Autodesk Inventor part; units mm, degrees
(part 4 of 4)
  line L2671 (9.6574, 16.9003) -> (9.6038, 16.7112)
  line L2672 (9.6038, 16.7112) -> (9.5545, 16.5545)
  line L2673 (9.5545, 16.5545) -> (9.5433, 16.503)
  line L2674 (9.5433, 16.503) -> (9.5383, 16.4584)
  line L2675 (9.5383, 16.4584) -> (9.5392, 16.4209)
  line L2676 (9.5392, 16.4209) -> (9.5457, 16.3908)
  line L2677 (9.5457, 16.3908) -> (9.5575, 16.3682)
  line L2678 (9.5575, 16.3682) -> (9.5743, 16.3534)
  line L2679 (9.5743, 16.3534) -> (9.6034, 16.3364)
  line L2680 (9.6034, 16.3364) -> (9.9014, 16.1575)
  line L2681 (9.9014, 16.1575) -> (10.196, 15.9733)
  line L2682 (10.196, 15.9733) -> (10.2244, 15.9551)
  line L2683 (10.2244, 15.9551) -> (10.2452, 15.9468)
  line L2684 (10.2452, 15.9468) -> (10.2706, 15.9466)
  line L2685 (10.2706, 15.9466) -> (10.3004, 15.9544)
  line L2686 (10.3004, 15.9544) -> (10.3342, 15.9707)
  line L2687 (10.3342, 15.9707) -> (10.3717, 15.9954)
  line L2688 (10.3717, 15.9954) -> (10.4125, 16.0287)
  line L2689 (10.4125, 16.0287) -> (10.5298, 16.1438)
  line L2690 (10.5298, 16.1438) -> (10.6739, 16.2774)
  line L2691 (10.6739, 16.2774) -> (10.8486, 16.4262)
  line L2692 (10.8486, 16.4262) -> (11.0549, 16.5875)
  line L2693 (11.0549, 16.5875) -> (11.2943, 16.7591)
  line L2694 (11.2943, 16.7591) -> (11.4265, 16.8478)
  line L2695 (11.4265, 16.8478) -> (11.5685, 16.9387)
  line L2696 (11.5685, 16.9387) -> (11.7175, 17.0299)
  line L2697 (11.7175, 17.0299) -> (11.8785, 17.1238)
  line L2698 (11.8785, 17.1238) -> (12.0338, 17.2101)
  arc A76 (12.6491, 16.763) -> (12.0338, 17.2101) centre (0, 0) ccw
  line L2699 (12.6491, 16.763) -> (12.615, 16.5887)
  line L2700 (12.615, 16.5887) -> (12.5755, 16.4066)
  line L2701 (12.5755, 16.4066) -> (12.5348, 16.2367)
  line L2702 (12.5348, 16.2367) -> (12.4922, 16.0735)
  line L2703 (12.4922, 16.0735) -> (12.4487, 15.9204)
  line L2704 (12.4487, 15.9204) -> (12.3595, 15.6397)
  line L2705 (12.3595, 15.6397) -> (12.2698, 15.3936)
  line L2706 (12.2698, 15.3936) -> (12.1823, 15.1815)
  line L2707 (12.1823, 15.1815) -> (12.0998, 15.0031)
  line L2708 (12.0998, 15.0031) -> (12.0266, 14.856)
  line L2709 (12.0266, 14.856) -> (12.0075, 14.8069)
  line L2710 (12.0075, 14.8069) -> (11.9956, 14.7636)
  line L2711 (11.9956, 14.7636) -> (11.9906, 14.7264)
  line L2712 (11.9906, 14.7264) -> (11.9923, 14.6957)
  line L2713 (11.9923, 14.6957) -> (12.0004, 14.6716)
  line L2714 (12.0004, 14.6716) -> (12.0147, 14.6544)
  line L2715 (12.0147, 14.6544) -> (12.0408, 14.633)
  line L2716 (12.0408, 14.633) -> (12.307, 14.4097)
  line L2717 (12.307, 14.4097) -> (12.5693, 14.1816)
  line L2718 (12.5693, 14.1816) -> (12.5944, 14.1592)
  line L2719 (12.5944, 14.1592) -> (12.6137, 14.1478)
  line L2720 (12.6137, 14.1478) -> (12.6388, 14.1436)
  line L2721 (12.6388, 14.1436) -> (12.6694, 14.1467)
  line L2722 (12.6694, 14.1467) -> (12.7053, 14.1574)
  line L2723 (12.7053, 14.1574) -> (12.7462, 14.1759)
  line L2724 (12.7462, 14.1759) -> (12.7918, 14.2025)
  line L2725 (12.7918, 14.2025) -> (12.9256, 14.2978)
  line L2726 (12.9256, 14.2978) -> (13.0888, 14.4072)
  line L2727 (13.0888, 14.4072) -> (13.2846, 14.5269)
  line L2728 (13.2846, 14.5269) -> (13.5137, 14.6539)
  line L2729 (13.5137, 14.6539) -> (13.777, 14.786)
  line L2730 (13.777, 14.786) -> (13.9214, 14.8528)
  line L2731 (13.9214, 14.8528) -> (14.0759, 14.9205)
  line L2732 (14.0759, 14.9205) -> (14.2373, 14.9872)
  line L2733 (14.2373, 14.9872) -> (14.411, 15.0547)
  line L2734 (14.411, 15.0547) -> (14.5779, 15.1157)
  arc A77 (15.1157, 14.5779) -> (14.5779, 15.1157) centre (0, 0) ccw
  line L2735 (15.1157, 14.5779) -> (15.0547, 14.411)
  line L2736 (15.0547, 14.411) -> (14.9872, 14.2373)
  line L2737 (14.9872, 14.2373) -> (14.9205, 14.0759)
  line L2738 (14.9205, 14.0759) -> (14.8529, 13.9214)
  line L2739 (14.8529, 13.9214) -> (14.786, 13.777)
  line L2740 (14.786, 13.777) -> (14.654, 13.5137)
  line L2741 (14.654, 13.5137) -> (14.5269, 13.2846)
  line L2742 (14.5269, 13.2846) -> (14.4072, 13.0888)
  line L2743 (14.4072, 13.0888) -> (14.2978, 12.9256)
  line L2744 (14.2978, 12.9256) -> (14.2025, 12.7918)
  line L2745 (14.2025, 12.7918) -> (14.1759, 12.7462)
  line L2746 (14.1759, 12.7462) -> (14.1574, 12.7053)
  line L2747 (14.1574, 12.7053) -> (14.1467, 12.6694)
  line L2748 (14.1467, 12.6694) -> (14.1436, 12.6387)
  line L2749 (14.1436, 12.6387) -> (14.1478, 12.6137)
  line L2750 (14.1478, 12.6137) -> (14.1592, 12.5944)
  line L2751 (14.1592, 12.5944) -> (14.1816, 12.5693)
  line L2752 (14.1816, 12.5693) -> (14.4097, 12.307)
  line L2753 (14.4097, 12.307) -> (14.633, 12.0408)
  line L2754 (14.633, 12.0408) -> (14.6544, 12.0147)
  line L2755 (14.6544, 12.0147) -> (14.6716, 12.0004)
  line L2756 (14.6716, 12.0004) -> (14.6957, 11.9923)
  line L2757 (14.6957, 11.9923) -> (14.7265, 11.9906)
  line L2758 (14.7265, 11.9906) -> (14.7636, 11.9956)
  line L2759 (14.7636, 11.9956) -> (14.8069, 12.0075)
  line L2760 (14.8069, 12.0075) -> (14.856, 12.0266)
  line L2761 (14.856, 12.0266) -> (15.0031, 12.0998)
  line L2762 (15.0031, 12.0998) -> (15.1815, 12.1823)
  line L2763 (15.1815, 12.1823) -> (15.3936, 12.2698)
  line L2764 (15.3936, 12.2698) -> (15.6397, 12.3595)
  line L2765 (15.6397, 12.3595) -> (15.9204, 12.4487)
  line L2766 (15.9204, 12.4487) -> (16.0735, 12.4922)
  line L2767 (16.0735, 12.4922) -> (16.2367, 12.5348)
  line L2768 (16.2367, 12.5348) -> (16.4066, 12.5755)
  line L2769 (16.4066, 12.5755) -> (16.5887, 12.615)
  line L2770 (16.5887, 12.615) -> (16.7631, 12.6491)
  arc A78 (17.2101, 12.0338) -> (16.7631, 12.6491) centre (0, 0) ccw
  line L2771 (17.2101, 12.0338) -> (17.1238, 11.8785)
  line L2772 (17.1238, 11.8785) -> (17.0299, 11.7175)
  line L2773 (17.0299, 11.7175) -> (16.9387, 11.5685)
  line L2774 (16.9387, 11.5685) -> (16.8478, 11.4265)
  line L2775 (16.8478, 11.4265) -> (16.7591, 11.2943)
  line L2776 (16.7591, 11.2943) -> (16.5875, 11.0549)
  line L2777 (16.5875, 11.0549) -> (16.4262, 10.8486)
  line L2778 (16.4262, 10.8486) -> (16.2774, 10.6739)
  line L2779 (16.2774, 10.6739) -> (16.1438, 10.5298)
  line L2780 (16.1438, 10.5298) -> (16.0287, 10.4125)
  line L2781 (16.0287, 10.4125) -> (15.9954, 10.3717)
  line L2782 (15.9954, 10.3717) -> (15.9707, 10.3342)
  line L2783 (15.9707, 10.3342) -> (15.9544, 10.3004)
  line L2784 (15.9544, 10.3004) -> (15.9466, 10.2706)
  line L2785 (15.9466, 10.2706) -> (15.9468, 10.2452)
  line L2786 (15.9468, 10.2452) -> (15.9551, 10.2244)
  line L2787 (15.9551, 10.2244) -> (15.9733, 10.196)
  line L2788 (15.9733, 10.196) -> (16.1575, 9.9013)
  line L2789 (16.1575, 9.9013) -> (16.3364, 9.6034)
  line L2790 (16.3364, 9.6034) -> (16.3535, 9.5743)
  line L2791 (16.3535, 9.5743) -> (16.3682, 9.5575)
  line L2792 (16.3682, 9.5575) -> (16.3908, 9.5457)
  line L2793 (16.3908, 9.5457) -> (16.4209, 9.5392)
  line L2794 (16.4209, 9.5392) -> (16.4584, 9.5383)
  line L2795 (16.4584, 9.5383) -> (16.503, 9.5433)
  line L2796 (16.503, 9.5433) -> (16.5545, 9.5545)
  line L2797 (16.5545, 9.5545) -> (16.7112, 9.6038)
  line L2798 (16.7112, 9.6038) -> (16.9003, 9.6574)
  line L2799 (16.9003, 9.6574) -> (17.1235, 9.7107)
  line L2800 (17.1235, 9.7107) -> (17.3806, 9.7608)
  line L2801 (17.3806, 9.7608) -> (17.6718, 9.805)
  line L2802 (17.6718, 9.805) -> (17.8299, 9.8239)
  line L2803 (17.8299, 9.8239) -> (17.9976, 9.8405)
  line L2804 (17.9976, 9.8405) -> (18.1718, 9.8541)
  line L2805 (18.1718, 9.8541) -> (18.3579, 9.8646)
  line L2806 (18.3579, 9.8646) -> (18.5354, 9.8711)
  arc A79 (18.8807, 9.1934) -> (18.5354, 9.8711) centre (0, 0) ccw
  line L2807 (18.8807, 9.1934) -> (18.7712, 9.0535)
  line L2808 (18.7712, 9.0535) -> (18.6532, 8.9092)
  line L2809 (18.6532, 8.9092) -> (18.5399, 8.7763)
  line L2810 (18.5399, 8.7763) -> (18.4279, 8.6503)
  line L2811 (18.4279, 8.6503) -> (18.3196, 8.5336)
  line L2812 (18.3196, 8.5336) -> (18.1127, 8.3239)
  line L2813 (18.1127, 8.3239) -> (17.9211, 8.1454)
  line L2814 (17.9211, 8.1454) -> (17.7468, 7.9961)
  line L2815 (17.7468, 7.9961) -> (17.5923, 7.8747)
  line L2816 (17.5923, 7.8747) -> (17.4603, 7.7769)
  line L2817 (17.4603, 7.7769) -> (17.4209, 7.7418)
  line L2818 (17.4209, 7.7418) -> (17.3907, 7.7086)
  line L2819 (17.3907, 7.7086) -> (17.3694, 7.6778)
  line L2820 (17.3694, 7.6778) -> (17.3569, 7.6496)
  line L2821 (17.3569, 7.6496) -> (17.3532, 7.6244)
  line L2822 (17.3532, 7.6244) -> (17.3581, 7.6026)
  line L2823 (17.3581, 7.6026) -> (17.3717, 7.5717)
  line L2824 (17.3717, 7.5717) -> (17.5075, 7.2518)
  line L2825 (17.5075, 7.2518) -> (17.6376, 6.9296)
  line L2826 (17.6376, 6.9296) -> (17.6499, 6.8982)
  line L2827 (17.6499, 6.8982) -> (17.6618, 6.8793)
  line L2828 (17.6618, 6.8793) -> (17.6823, 6.8641)
  line L2829 (17.6823, 6.8641) -> (17.711, 6.853)
  line L2830 (17.711, 6.853) -> (17.7479, 6.8462)
  line L2831 (17.7479, 6.8462) -> (17.7927, 6.8442)
  line L2832 (17.7927, 6.8442) -> (17.8454, 6.8472)
  line L2833 (17.8454, 6.8472) -> (18.0079, 6.8714)
  line L2834 (18.0079, 6.8714) -> (18.203, 6.8947)
  line L2835 (18.203, 6.8947) -> (18.4318, 6.9124)
  line L2836 (18.4318, 6.9124) -> (18.6935, 6.9217)
  line L2837 (18.6935, 6.9217) -> (18.9881, 6.9198)
  line L2838 (18.9881, 6.9198) -> (19.1472, 6.9138)
  line L2839 (19.1472, 6.9138) -> (19.3155, 6.9039)
  line L2840 (19.3155, 6.9039) -> (19.4896, 6.8901)
  line L2841 (19.4896, 6.8901) -> (19.675, 6.8714)
  line L2842 (19.675, 6.8714) -> (19.8514, 6.85)
  arc A80 (20.0864, 6.1266) -> (19.8514, 6.85) centre (0, 0) ccw
  line L2843 (20.0864, 6.1266) -> (19.9563, 6.0056)
  line L2844 (19.9563, 6.0056) -> (19.8173, 5.8815)
  line L2845 (19.8173, 5.8815) -> (19.6846, 5.7679)
  line L2846 (19.6846, 5.7679) -> (19.5542, 5.661)
  line L2847 (19.5542, 5.661) -> (19.429, 5.5627)
  line L2848 (19.429, 5.5627) -> (19.1918, 5.388)
  line L2849 (19.1918, 5.388) -> (18.9746, 5.2416)
  line L2850 (18.9746, 5.2416) -> (18.7791, 5.1215)
  line L2851 (18.7791, 5.1215) -> (18.6076, 5.0257)
  line L2852 (18.6076, 5.0257) -> (18.4619, 4.9497)
  line L2853 (18.4619, 4.9497) -> (18.4175, 4.9212)
  line L2854 (18.4175, 4.9212) -> (18.3824, 4.8932)
  line L2855 (18.3824, 4.8932) -> (18.3566, 4.8661)
  line L2856 (18.3566, 4.8661) -> (18.3399, 4.8402)
  line L2857 (18.3399, 4.8402) -> (18.3323, 4.8159)
  line L2858 (18.3323, 4.8159) -> (18.3337, 4.7936)
  line L2859 (18.3337, 4.7936) -> (18.3423, 4.761)
  line L2860 (18.3423, 4.761) -> (18.4264, 4.4238)
  line L2861 (18.4264, 4.4238) -> (18.5045, 4.0851)
  line L2862 (18.5045, 4.0851) -> (18.5117, 4.0522)
  line L2863 (18.5117, 4.0522) -> (18.5205, 4.0317)
  line L2864 (18.5205, 4.0317) -> (18.5383, 4.0135)
  line L2865 (18.5383, 4.0135) -> (18.565, 3.998)
  line L2866 (18.565, 3.998) -> (18.6003, 3.9856)
  line L2867 (18.6003, 3.9856) -> (18.6443, 3.9765)
  line L2868 (18.6443, 3.9765) -> (18.6968, 3.9713)
  line L2869 (18.6968, 3.9713) -> (18.8611, 3.9697)
  line L2870 (18.8611, 3.9697) -> (19.0574, 3.9623)
  line L2871 (19.0574, 3.9623) -> (19.2862, 3.944)
  line L2872 (19.2862, 3.944) -> (19.5462, 3.9122)
  line L2873 (19.5462, 3.9122) -> (19.8368, 3.8642)
  line L2874 (19.8368, 3.8642) -> (19.993, 3.8334)
  line L2875 (19.993, 3.8334) -> (20.1577, 3.7973)
  line L2876 (20.1577, 3.7973) -> (20.3275, 3.7564)
  line L2877 (20.3275, 3.7564) -> (20.5077, 3.7089)
  line L2878 (20.5077, 3.7089) -> (20.6786, 3.6602)
  arc A81 (20.7975, 2.909) -> (20.6786, 3.6602) centre (0, 0) ccw
  line L2879 (20.7975, 2.909) -> (20.6501, 2.8098)
  point P0 (0, 0)
  constraints: 5760 end point, 720 perpendicular, 360 parallel, 4 horizontal alignment, 4 vertical alignment, 235 other
extrude "Extrusion1" add sketch "Sketch4" along normal blind 6.2
sketch "Sketch5" plane through (0, 0, 0) normal (0, 0, -1) x (-1, 0, 0)
  circle A0 centre (0, 0) radius 2 projected
  line L0 (0, 0) -> (3.1, 0) construction
  line L1 (0, 0) -> (1.55, 2.6847) construction
  line L2 (0, 0) -> (-1.55, 2.6847) construction
  line L3 (0, 0) -> (-3.1, 0) construction
  line L4 (0, 0) -> (-1.55, -2.6847) construction
  line L5 (0, 0) -> (1.55, -2.6847) construction
  line L6 (-1.55, 2.6847) -> (1.55, 2.6847)
  line L7 (1.55, 2.6847) -> (3.1, 0)
  line L8 (1.55, -2.6847) -> (-1.55, -2.6847)
  line L9 (-1.55, -2.6847) -> (-3.1, 0)
  line L10 (-1.55, 2.6847) -> (-3.1, 0)
  line L11 (1.55, -2.6847) -> (3.1, 0)
  line L12 (3.6773, 0) -> (1.8387, 3.1847)
  line L13 (1.8387, 3.1847) -> (-1.8387, 3.1847)
  line L14 (-1.8387, 3.1847) -> (-3.6774, 0)
  line L15 (-3.6774, 0) -> (-1.8387, -3.1847)
  line L16 (-1.8387, -3.1847) -> (1.8387, -3.1847)
  line L17 (1.8387, -3.1847) -> (3.6773, 0)
  point P0 (0, 0)
  dimension "d7" = 3.1
  dimension "d10" = 360
  dimension "d14" = 0.5
  constraints: 36 end point, 6 parallel, 2 coincident, 2 horizontal, 22 other
  measures "d7" distance of L0.start L0.end
  measures "d14" distance between parallel lines of L11 L17
extrude "Extrusion2" cut sketch "Sketch5" against normal blind 6.2 contours A0 | L6 L7 L11 L8 L9 L10 | L17 L16 L15 L14 L13 L12
body "Solid1"
